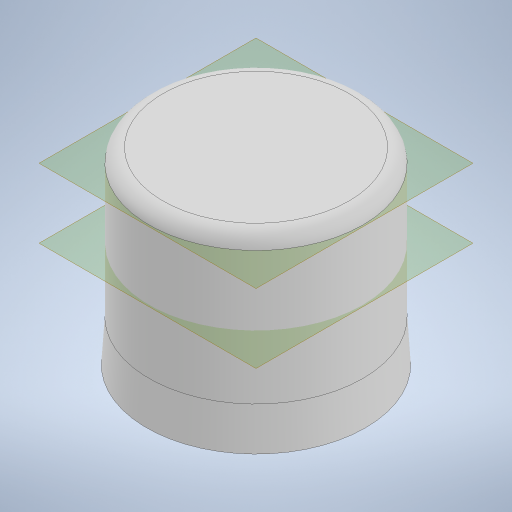
# Autodesk Inventor part: Pope8697-Lid
Saved by Autodesk Inventor 2023 (Build 270158000, 158)
## iProperties
Created: 2024-07-11
Part Number: Pope8697-Lid
Material: Generic
Document SubType Name: Modeling
Designer: incep
Density: 1 g/cm^3
Appearance: Default
Author: incep
## iProperties of the stored document Pope8697-Adapter_3DPrint.ipt
Created: 2024-07-10
Part Number: Pope8697-Adapter_3DPrint
Material: Generic
Document SubType Name: Modeling
Designer: incep
Density: 1 g/cm^3
Appearance: Default
Author: incep
Autodesk Inventor part; units mm, degrees
ref_plane "YZ Plane" through (0, 0, 0) normal (1, 0, 0) x (0, 1, 0)
sketch "Sketch1" plane through (0, 0, 0) normal (0, 1, 0) x (-1, 0, 0)
  circle A0 centre (0, 0) radius 35.1 construction
  circle A1 centre (0, 0) radius 31.4 construction
  circle A2 centre (0, 0) radius 36 construction
  circle A3 centre (0, 0) radius 27.65 construction
  circle A4 centre (0, 0) radius 32.3 construction
  circle A5 centre (0, 0) radius 31.8
  circle A6 centre (0, 0) radius 36.5
  circle A7 centre (0, 0) radius 29.8
  circle A8 centre (0, 0) radius 39.5
  dimension "d0" = 70.2
  dimension "d1" = 62.8
  dimension "d2" = 72
  dimension "d3" = 55.3
  dimension "d4" = 0.9
  dimension "d5" = 0.9
  dimension "d6" = 0.5
  dimension "d7" = 0.5
  dimension "d11" = 2
  dimension "d12" = 3
  constraints: 9 centre point, 4 coincident
  measures "d0" diameter of A0
  measures "d1" diameter of A1
  measures "d2" diameter of A2
  measures "d3" diameter of A3
  measures "d4" radial gap between concentric circles of A2 A0
  measures "d5" radial gap between concentric circles of A1 A4
  measures "d6" radial gap between concentric circles of A4 A5
  measures "d7" radial gap between concentric circles of A2 A6
  measures "d11" radial gap between concentric circles of A5 A7
  measures "d12" radial gap between concentric circles of A6 A8
ref_plane "Work Plane1" through (0, 15, 0) normal (0, 1, 0) x (-1, 0, 0)
sketch "Sketch2" plane through (0, 15, 0) normal (0, 1, 0) x (-1, 0, 0)
  circle A0 centre (0, 0) radius 35.1 construction
  circle A1 centre (0, 0) radius 31.4 construction
  circle A2 centre (0, 0) radius 35.6
  circle A3 centre (0, 0) radius 30.9
  circle A4 centre (0, 0) radius 38.6
  circle A5 centre (0, 0) radius 28.9
  dimension "d9" = 0.5
  dimension "d10" = 0.5
  dimension "d13" = 3
  dimension "d14" = 2
  constraints: 4 centre point
  measures "d9" radial gap between concentric circles of A0 A2
  measures "d10" radial gap between concentric circles of A1 A3
  measures "d13" radial gap between concentric circles of A2 A4
  measures "d14" radial gap between concentric circles of A3 A5
loft "Loft1" add profiles "Sketch2", "Sketch1" contours A2 | A3 | A4 | A5 / A5 | A6 | A7 | A8
loft "Loft2" cut profiles "Sketch1", "Sketch2" contours A5 | A6 | A7 / A2 | A3 | A5
extrude "Extrusion1" add sketch "Sketch2" against normal up to surface (15 mm away) contours A3
sketch "Sketch3" plane through (0, 15, 0) normal (0, 1, 0) x (1, 0, 0)
  circle A0 centre (0, 0) radius 38.6 projected
  circle A1 centre (0, 0) radius 28.9 projected
  circle A2 centre (0, 0) radius 60.865
  dimension "d27" = 121.73
  constraints: 1 centre point, 1 coincident
  measures "d27" diameter of A2
extrude "Extrusion2" add sketch "Sketch3" along normal blind 3 contours A0
ref_plane "Mating Plane with Cooling Shroud" through (0, 72.6, 0) normal (0, -1, 0) x (1, 0, 0)
ref_plane "Plane of the K flange face" through (0, 39, 0) normal (0, -1, 0) x (1, 0, 0)
sketch "Sketch4" plane through (0, 0, 0) normal (0, 1, 0) x (1, 0, 0)
  circle A0 centre (0, 0) radius 55 construction
  circle A1 centre (0, 55) radius 2.9
  circle A2 centre (0, 0) radius 39.5 construction
  circle A3 centre (0, 0) radius 60.865
  circle A4 centre (0, 0) radius 39.5 projected
  circle A5 centre (0, 0) radius 36.5 projected
  dimension "d30" = 110
  dimension "d31" = 5.8
  dimension "d32" = 121.73
  constraints: 2 centre point, 2 coincident, 1 vertical alignment, 2 other
  measures "d31" diameter of A1
  measures "d32" diameter of A3
extrude "Extrusion3" [suppressed]
extrude "Extrusion4" [suppressed]
pattern_circular "Circular Pattern1" [suppressed]
sketch "Sketch5" plane through (0, 18, 0) normal (0, 1, 0) x (1, 0, 0)
  circle A0 centre (0, 0) radius 28.9 projected
  circle A1 centre (0, 0) radius 31.9
  dimension "d40" = 3
  constraints: 1 centre point
  measures "d40" radial gap between concentric circles of A0 A1
extrude "Extrusion5" [suppressed]
sketch "Sketch7" plane through (0, 0, 0) normal (1, 0, 0) x (0, 1, 0)
  line L0 (0, -60.865) -> (3, -60.865) projected
  line L1 (3, -60.865) -> (3, 60.865) projected
  line L2 (0, -39.5) -> (15, -38.6) projected
  line L3 (15, -38.6) -> (18, -38.6) projected
  line L4 (18, -38.6) -> (18, 38.6) projected
  line L5 (18, -31.9) -> (72.6, -31.9) projected
  line L6 (3, -60.865) -> (72.6, -60.865)
  line L7 (72.6, -60.865) -> (72.6, -31.9)
  line L8 (-14.1, 0) -> (84.6, 0) projected
  point P0 (0, 0)
  constraints: 4 end point, 1 horizontal, 1 perpendicular, 1 other
revolve "Revolution1" [suppressed]
pattern_circular "Circular Pattern2" [suppressed]
extrude "Extrusion6" [suppressed]
pattern_circular "Circular Pattern3" [suppressed]
sketch "Sketch8" plane through (0, 72.6, 0) normal (0, 1, 0) x (-1, 0, 0)
  circle A0 centre (0, 0) radius 39.85
  point P0 (0, 0)
  dimension "d52" = 79.7
  constraints: 1 centre point, 1 coincident
  measures "d52" diameter of A0
extrude "Extrusion7" [suppressed]
sketch "Sketch9" plane through (0, 55.6, 0) normal (0, 1, 0) x (1, 0, 0)
  circle A0 centre (0, 0) radius 19.55
  arc A1 (-24.4368, -20.5049) -> (24.4368, -20.5049) centre (0, 0) ccw projected
  circle A2 centre (0, 0) radius 31.9
  point P0 (-24.4368, -20.5049)
  dimension "d57" = 39.1
  constraints: 2 centre point, 1 coincident, 1 concentric
  measures "d57" diameter of A0
extrude "Extrusion8" [suppressed]
sketch "Sketch10" plane through (0, 57.6, 0) normal (0, 1, 0) x (1, 0, 0)
  arc A0 (6, -25.55) -> (-6, -25.55) centre (0, -25.55) ccw
  line L0 (-6, -31.9) -> (6, -31.9) construction
  circle A1 centre (0, 0) radius 31.9 projected
  line L1 (-6, -31.9) -> (-6, -25.55)
  line L2 (6, -31.9) -> (6, -25.55)
  circle A2 centre (0, 0) radius 19.55 projected
  point P0 (0, -31.9)
  point P1 (-6, -31.3307)
  point P2 (6, -31.3307)
  dimension "d58" = 12
  dimension "d60" = 12
  constraints: 6 end point, 4 tangent, 2 point on circle, 2 vertical alignment, 1 centre point, 1 horizontal, 1 midpoint
  measures "d58" diameter of A0
  measures "d60" distance of L0.start L0.end
extrude "Extrusion9" [suppressed]
ref_plane "Work Plane4" through (0, 67.6, 31.9) normal (0, 0, 1) x (1, 0, 0)
sketch "Sketch11" plane through (0, 67.6, 31.9) normal (0, 0, 1) x (1, 0, 0)
  circle A0 centre (0, -5) radius 3.85
  line L0 (6, 0) -> (-6, 0) projected
  line L1 (-6, -10) -> (-6, 0) projected
  point P0 (0, -67.6)
  point P1 (0, 0)
  point P2 (-6, -5)
  dimension "d63" = 7.7
  constraints: 2 midpoint, 1 centre point, 1 horizontal alignment, 1 vertical alignment
  measures "d63" diameter of A0
extrude "Extrusion10" [suppressed]
sketch "Sketch12" plane through (0, 67.6, 0) normal (0, 1, 0) x (1, 0, 0)
  point P0 (0, 0)
sketch "Sketch13" plane through (0, 62.6, 22.9) normal (0, 0, 1) x (1, 0, 0)
  circle A0 centre (0, 0) radius 0.75
  point P0 (0, -62.6)
  dimension "d66" = 1.5
  constraints: 1 centre point
  measures "d66" diameter of A0
extrude "Extrusion11" [suppressed]
sketch "Sketch15" plane through (0, 55.6, 0) normal (0, -1, 0) x (1, 0, 0)
  line L0 (-3.85, 22.9) -> (3.85, 22.9) projected
  circle A0 centre (0, 22.9) radius 1.5
  point P0 (0, 0)
  point P1 (-0.75, 22.9)
  point P2 (0.75, 22.9)
  dimension "d71" = 3
  constraints: 1 centre point, 1 midpoint
  measures "d71" diameter of A0
ref_plane "Work Plane5" through (0, 66.45, 31.9) normal (0, 1, 0) x (-1, 0, 0)
extrude "Extrusion12" [suppressed]
sketch "Sketch16" plane through (0, 57.6, 0) normal (0, 1, 0) x (1, 0, 0)
  line L0 (-19.55, 0) -> (-19.55, -35)
  line L1 (-19.55, -35) -> (19.55, -35)
  line L2 (19.55, -35) -> (19.55, 0)
  circle A0 centre (0, 0) radius 19.55 projected
  line L3 (-19.05, 0) -> (-19.05, -35)
  line L4 (19.05, 0) -> (19.05, -35)
  line L5 (-19.55, 0) -> (19.55, 0)
  point P0 (19.55, 0)
  point P1 (-19.05, -4.3932)
  point P2 (19.05, -4.3932)
  dimension "d74" = 0.5
  dimension "d75" = 0.5
  dimension "d76" = 35
  constraints: 12 end point, 4 perpendicular, 2 point on circle, 2 point on line, 2 tangent, 1 horizontal, 1 vertical
  measures "d74" distance between parallel lines of L0 L3
  measures "d75" distance between parallel lines of L2 L4
  measures "d76" distance of L0.start L0.end
extrude "Extrusion13" [suppressed]
ref_plane "Inside Plane of Lid Top" through (0, 63, 0) normal (0, -1, 0) x (1, 0, 0)
ref_plane "Top of the Dewar Neck" through (0, 38, 0) normal (0, -1, 0) x (1, 0, 0)
sketch "Sketch18" plane through (0, 18, 0) normal (0, 1, 0) x (1, 0, 0)
  circle A0 centre (0, 0) radius 38.6 projected
  circle A1 centre (0, 0) radius 28.9 projected
extrude "Extrusion14" add sketch "Sketch18" along normal up to surface (45 mm away)
sketch "Sketch19" plane through (0, 63, 0) normal (0, 1, 0) x (1, 0, 0)
  circle A0 centre (0, 0) radius 38.6 projected
extrude "Extrusion15" add sketch "Sketch19" along normal blind 5
fillet "Fillet1" radius 5 1 edges at (-38.6, 68, 0)
fillet "Fillet2" radius 5 1 edges at (-28.9, 63, 0)
body "Solid1"
body "Solid2"
